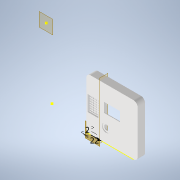
# Autodesk Inventor part: PCB_Deckel
Saved by Autodesk Inventor 2022.2 (Build 262287010, 287A)
## iProperties
Created: 2022-02-22
Part Number: PCB_Deckel
Material: Generisch
Document SubType Name: Modeling
Designer: hpcwoess
Density: 1 g/cm^3
Appearance: Vorgabe
Author: hpcwoess
Autodesk Inventor part; units mm, degrees
ref_plane "YZ Plane" through (0, 0, 0) normal (1, 0, 0) x (0, 1, 0)
ref_plane "XZ Plane" through (0, 0, 0) normal (0, 1, 0) x (-1, 0, 0)
ref_plane "Arbeitsebene1" through (0, 0, 9) normal (0, 0, 1) x (1, 0, 0)
sketch "Skizze1" plane through (0, 0, 9) normal (0, 0, 1) x (1, 0, 0)
  line L0 (68, -33.7) -> (131, -33.7)
  arc A0 (135.4, -38.1) -> (131, -33.7) centre (131, -38.1) ccw
  line L1 (135.4, -38.1) -> (135.4, -101.1)
  arc A1 (131, -105.5) -> (135.4, -101.1) centre (131, -101.1) ccw
  line L2 (131, -105.5) -> (68, -105.5)
  arc A2 (63.6, -101.1) -> (68, -105.5) centre (68, -101.1) ccw
  line L3 (63.6, -101.1) -> (63.6, -38.1)
  arc A3 (68, -33.7) -> (63.6, -38.1) centre (68, -38.1) ccw
  line L4 (131, -31.7) -> (68, -31.7)
  arc A4 (68, -31.7) -> (61.6, -38.1) centre (68, -38.1) ccw
  line L5 (61.6, -38.1) -> (61.6, -101.1)
  arc A5 (61.6, -101.1) -> (68, -107.5) centre (68, -101.1) ccw
  line L6 (68, -107.5) -> (131, -107.5)
  arc A6 (131, -107.5) -> (137.4, -101.1) centre (131, -101.1) ccw
  line L7 (137.4, -101.1) -> (137.4, -38.1)
  arc A7 (137.4, -38.1) -> (131, -31.7) centre (131, -38.1) ccw
  circle A8 centre (90.798, -87.67) radius 3.75
  line L8 (87.5, -55.7) -> (111.5, -55.7)
  line L9 (111.5, -55.7) -> (111.5, -69.7)
  line L10 (111.5, -69.7) -> (87.5, -69.7)
  line L11 (87.5, -69.7) -> (87.5, -55.7)
  circle A9 centre (73.806, -50.504) radius 4.35
  circle A10 centre (73.806, -87.588) radius 4.35
  point P0 (0, 0)
  point P1 (99.5, -55.7)
  dimension "d2" = 2
  dimension "d3" = 7.5
  dimension "d6" = 24
  dimension "d7" = 14
  dimension "d8" = 71.8
  dimension "d9" = 23.9
  dimension "d10" = 22
  constraints: 24 end point, 16 point on circle, 11 centre point, 2 parallel, 1 horizontal, 1 midpoint, 1 perpendicular, 7 other
  measures "d2" distance between parallel lines of L0 L4
  measures "d3" diameter of A8
  measures "d6" distance of L9.end L10.end
  measures "d7" distance of L8.end L9.end
  measures "d8" distance between parallel lines of L1 L3
  measures "d9" distance between parallel lines of L11 L3
  measures "d10" distance from line of point (99.5, -55.7) L0
extrude "Extrusion1" add sketch "Skizze1" along normal blind 2 contours L0 A0 L1 A1 L2 A2 L3 A3 | A7 L7 A6 L6 A5 L5 A4 L4 | A9 | A10
sketch "Skizze2" plane through (0, 0, 9) normal (0, 0, -1) x (-1, 0, 0)
  line L0 (-61.6, -38.1) -> (-61.6, -101.1) projected
  arc A0 (-61.6, -38.1) -> (-68, -31.7) centre (-68, -38.1) ccw projected
  line L1 (-131, -31.7) -> (-68, -31.7) projected
  arc A1 (-131, -31.7) -> (-137.4, -38.1) centre (-131, -38.1) ccw projected
  line L2 (-137.4, -101.1) -> (-137.4, -38.1) projected
  arc A2 (-137.4, -101.1) -> (-131, -107.5) centre (-131, -101.1) ccw projected
  line L3 (-68, -107.5) -> (-131, -107.5) projected
  arc A3 (-68, -107.5) -> (-61.6, -101.1) centre (-68, -101.1) ccw projected
  line L4 (-63.6, -101.1) -> (-63.6, -38.1)
  arc A4 (-63.6, -38.1) -> (-68, -33.7) centre (-68, -38.1) ccw
  line L5 (-68, -33.7) -> (-131, -33.7)
  arc A5 (-131, -33.7) -> (-135.4, -38.1) centre (-131, -38.1) ccw
  line L6 (-135.4, -38.1) -> (-135.4, -101.1)
  arc A6 (-135.4, -101.1) -> (-131, -105.5) centre (-131, -101.1) ccw
  line L7 (-131, -105.5) -> (-68, -105.5)
  arc A7 (-68, -105.5) -> (-63.6, -101.1) centre (-68, -101.1) ccw
  point P0 (0, 0)
  dimension "d15" = 2
  constraints: 8 end point, 8 point on circle, 4 centre point, 7 other
  measures "d15" distance between parallel lines of L0 L4
extrude "Extrusion2" add sketch "Skizze2" along normal blind 9
sketch "Skizze3" plane through (87.5, -55.7, 9) normal (0, -1, 0) x (1, 0, 0)
  line L0 (-19.5, 0) -> (43.5, 0) projected
  line L1 (-5.6, 0) -> (-4, 0)
  line L2 (-4, 0) -> (-4, -7.3)
  line L3 (-4, -7.3) -> (-5.6, -7.3)
  line L4 (-5.6, -7.3) -> (-5.6, 0)
  line L5 (-23.9, 0) -> (-23.9, -9) projected
  point P0 (-87.5, -9)
  point P1 (-4, 0)
  dimension "d18" = 1.6
  dimension "d19" = 18.3
  dimension "d20" = 7.3
  constraints: 8 end point, 2 parallel, 1 horizontal, 1 perpendicular, 1 point on line
  measures "d18" distance of L2.end L3.end
  measures "d19" distance between parallel lines of L5 L4
  measures "d20" distance of L3.end L1.start
extrude "Extrusion3" add sketch "Skizze3" along normal blind 51.75 and the other way blind 24
sketch "Skizze4" plane through (0, 0, 9) normal (0, 0, -1) x (-1, 0, 0)
  line L0 (-131, -33.7) -> (-68, -33.7) projected
  arc A0 (-63.6, -38.1) -> (-68, -33.7) centre (-68, -38.1) ccw projected
  line L1 (-63.6, -38.1) -> (-63.6, -101.1) projected
  arc A1 (-68, -105.5) -> (-63.6, -101.1) centre (-68, -101.1) ccw projected
  line L2 (-68, -105.5) -> (-131, -105.5) projected
  line L3 (-81.9, -33.7) -> (-81.9, -105.5) projected
  line L4 (-81.9, -33.7) -> (-81.9, -105.5) projected
  line L5 (-81.9, -33.7) -> (-81.9, -105.5)
  line L6 (-81.9, -105.5) -> (-68, -105.5)
  line L7 (-63.6, -58.7) -> (-81.9, -58.7)
  line L8 (-63.6, -79.5) -> (-81.9, -79.5)
  circle A2 centre (-73.806, -50.504) radius 4.35 projected
  circle A3 centre (-73.806, -87.588) radius 4.35 projected
  point P0 (0, 0)
  dimension "d25" = 25
  dimension "d26" = 26
  constraints: 8 end point, 4 point on line, 2 perpendicular, 1 collinear, 1 vertical
  measures "d25" distance from line of L0 L7.end
  measures "d26" distance from line of L8.end L2
extrude "Extrusion4" add sketch "Skizze4" along normal blind 2.75 contours L0 A0 L1 L7 L3 | L8 L1 A1 L2 L3
sketch "Skizze5" plane through (0, 0, 6.25) normal (0, 0, -1) x (-1, 0, 0)
  line L0 (-81.9, -58.7) -> (-63.6, -58.7) projected
  line L1 (-81.9, -33.7) -> (-81.9, -105.5) projected
  line L2 (-63.6, -58.7) -> (-81.9, -58.7)
  line L3 (-81.9, -58.7) -> (-81.9, -56.7)
  line L4 (-81.9, -56.7) -> (-63.6, -56.7)
  line L5 (-63.6, -56.7) -> (-63.6, -58.7)
  line L6 (-63.6, -79.5) -> (-63.6, -101.1) projected
  line L7 (-63.6, -79.5) -> (-81.9, -79.5)
  line L8 (-81.9, -79.5) -> (-81.9, -81.5)
  line L9 (-81.9, -81.5) -> (-63.6, -81.5)
  line L10 (-63.6, -81.5) -> (-63.6, -79.5)
  point P0 (0, 0)
  dimension "d29" = 2
  dimension "d30" = 2
  constraints: 16 end point, 4 parallel, 2 horizontal, 2 perpendicular, 2 point on line
  measures "d29" distance between parallel lines of L9 L7
  measures "d30" distance between parallel lines of L0 L4
extrude "Extrusion5" add sketch "Skizze5" along normal up to surface (4.55 mm away)
sketch "Skizze6" plane through (68, -107.5, 11) normal (0, -1, 0) x (1, 0, 0)
  line L0 (-4.4, -4.75) -> (13.9, -4.75) projected
  line L1 (13.9, -4.75) -> (13.9, -4.75) projected
  line L2 (0, -4.75) -> (13.9, -4.75) projected
  line L3 (-4.4, -4.75) -> (0, -4.75) projected
  line L4 (-4.4, -4.75) -> (-4.4, -4.75) projected
  line L5 (10.156, -4.75) -> (1.456, -4.75) projected
  line L6 (-6.4, -11) -> (-6.4, 0) projected
  line L7 (-6.4, -2.75) -> (12.85, -2.75)
  line L8 (63, 0) -> (0, 0) projected
  arc A0 (12.85, -2.75) -> (15.6, 0) centre (12.85, 0) ccw
  line L9 (-6.4, -2.75) -> (-6.4, 0)
  line L10 (0, 0) -> (-6.4, 0) projected
  line L11 (15.6, 0) -> (0, 0)
  line L12 (0, 0) -> (63, 0) projected
  point P0 (-68, -11)
  point P1 (5.806, -4.75)
  dimension "d33" = 2
  dimension "d102" = 22
  constraints: 6 end point, 2 horizontal, 2 point on circle, 2 point on line, 1 centre point, 1 collinear, 1 line through centre, 1 midpoint, 1 tangent
  measures "d33" distance from line of L7 point (5.806, -4.75)
  measures "d102" distance from line of L11.start L6
ref_plane "Arbeitsebene2" through (81.9, -81.5, 1.7) normal (1, 0, 0) x (0, 1, 0)
sketch "Skizze9" plane through (81.9, -81.5, 1.7) normal (1, 0, 0) x (0, 1, 0)
  line L0 (-24, 0) -> (47.8, 0) projected
  line L1 (18.0018, 0) -> (13.8035, 0)
  line L2 (13.8035, 0) -> (13.8035, 1.2366)
  line L3 (13.8035, 1.2366) -> (18.0018, 1.2366)
  line L4 (18.0018, 1.2366) -> (18.0018, 0)
  line L5 (-16.9587, 0) -> (-21.7715, 0)
  line L6 (-21.7715, 0) -> (-21.7715, 0.4193)
  line L7 (-21.7715, 0.4193) -> (-16.9587, 0.4193)
  line L8 (-16.9587, 0.4193) -> (-16.9587, 0)
  point P0 (81.5, -1.7)
  constraints: 16 end point, 4 parallel, 2 horizontal, 2 perpendicular, 2 point on line
extrude "Extrusion8" cut sketch "Skizze9" along normal blind 10
ref_plane "Arbeitsebene4" through (68, -107.5, 8.25) normal (0, 0, 1) x (1, 0, 0)
sketch "Skizze10" plane through (68, -107.5, 11) normal (0, 0, 1) x (1, 0, 0)
  line L0 (-4.4, 69.4) -> (-4.4, 6.4) projected
  line L1 (-4.4, 49.8) -> (11.6, 49.8)
  line L2 (11.6, 49.8) -> (11.6, 26.8)
  line L3 (11.6, 26.8) -> (-4.4, 26.8)
  line L4 (-4.4, 26.8) -> (-4.4, 49.8)
  line L5 (12.85, 48.8) -> (-4.4, 48.8) projected
  point P0 (-68, 107.5)
  point P1 (13.9021, 48.8)
  point P2 (-4.4, 26.8)
  dimension "d43" = 16
  dimension "d44" = 23
  dimension "d45" = 1
  constraints: 8 end point, 2 parallel, 1 horizontal, 1 perpendicular, 1 point on line
  measures "d43" distance of L2.end L3.end
  measures "d44" distance of L1.end L2.end
  measures "d45" distance from line of L1.start L5
extrude "Extrusion9" cut sketch "Skizze10" against normal blind 2
ref_plane "Arbeitsebene3" through (68, -107.5, 8.25) normal (0, 0, 1) x (1, 0, 0)
sketch "Skizze11" plane through (68, -107.5, 11) normal (0, 0, 1) x (1, 0, 0)
  line L0 (11.6, 48.8) -> (13.9, 48.8) projected
  line L1 (13.9, 28) -> (11.6, 28) projected
  line L2 (12.5525, 48.8) -> (11.6, 48.8)
  line L3 (11.6, 48.8) -> (11.6, 28)
  line L4 (11.6, 28) -> (12.5525, 28)
  line L5 (12.5525, 28) -> (12.5525, 48.8)
  point P0 (-68, 107.5)
  point P1 (11.6, 48.8)
  point P2 (12.5525, 28)
  constraints: 8 end point, 2 parallel, 1 horizontal, 1 perpendicular, 1 point on line
extrude "Extrusion10" add sketch "Skizze11" against normal up to surface (9.3 mm away)
ref_plane "Arbeitsebene5" through (68, -107.5, 8.25) normal (0, 0, 1) x (1, 0, 0)
sketch "Skizze12" plane through (68, -107.5, 8.25) normal (0, 0, 1) x (1, 0, 0)
  line L0 (11.6, 49.8) -> (-4.4, 49.8) projected
  line L1 (-4.4, 26.8) -> (11.6, 26.8) projected
  line L2 (10.4, 49.8) -> (9.2, 49.8)
  line L3 (9.2, 49.8) -> (9.2, 26.8)
  line L4 (9.2, 26.8) -> (10.4, 26.8)
  line L5 (10.4, 26.8) -> (10.4, 49.8)
  line L6 (11.6, 49.8) -> (11.6, 26.8) projected
  line L7 (8, 49.8) -> (6.8, 49.8)
  line L8 (6.8, 49.8) -> (6.8, 26.8)
  line L9 (6.8, 26.8) -> (8, 26.8)
  line L10 (8, 26.8) -> (8, 49.8)
  line L11 (5.6, 49.8) -> (4.4, 49.8)
  line L12 (4.4, 49.8) -> (4.4, 26.8)
  line L13 (4.4, 26.8) -> (5.6, 26.8)
  line L14 (5.6, 26.8) -> (5.6, 49.8)
  line L15 (3.2, 49.8) -> (2, 49.8)
  line L16 (2, 49.8) -> (2, 26.8)
  line L17 (2, 26.8) -> (3.2, 26.8)
  line L18 (3.2, 26.8) -> (3.2, 49.8)
  line L19 (0.8, 49.8) -> (-0.4, 49.8)
  line L20 (-0.4, 49.8) -> (-0.4, 26.8)
  line L21 (-0.4, 26.8) -> (0.8, 26.8)
  line L22 (0.8, 26.8) -> (0.8, 49.8)
  line L23 (-1.6, 49.8) -> (-2.8, 49.8)
  line L24 (-2.8, 49.8) -> (-2.8, 26.8)
  line L25 (-2.8, 26.8) -> (-1.6, 26.8)
  line L26 (-1.6, 26.8) -> (-1.6, 49.8)
  line L27 (-4, 49.8) -> (-5.2, 49.8)
  line L28 (-5.2, 49.8) -> (-5.2, 26.8)
  line L29 (-5.2, 26.8) -> (-4, 26.8)
  line L30 (-4, 26.8) -> (-4, 49.8)
  point P0 (-68, 107.5)
  point P1 (-1.6, 49.8)
  point P2 (-2.8, 49.8)
  point P3 (-2.8, 26.8)
  point P4 (0.8, 26.8)
  point P5 (0.8, 49.8)
  point P6 (-0.4, 49.8)
  point P7 (-0.4, 26.8)
  point P8 (3.2, 26.8)
  point P9 (3.2, 49.8)
  point P10 (2, 49.8)
  point P11 (2, 26.8)
  point P12 (5.6, 26.8)
  point P13 (5.6, 49.8)
  point P14 (4.4, 49.8)
  point P15 (4.4, 26.8)
  point P16 (8, 49.8)
  point P17 (6.8, 49.8)
  point P18 (6.8, 26.8)
  point P19 (10.4, 26.8)
  point P20 (9.2, 49.8)
  dimension "d50" = 1.2
  dimension "d51" = 1.2
  dimension "d54" = 2.4
  constraints: 56 end point, 2 horizontal, 2 parallel, 2 point on line, 1 perpendicular, 48 other
  measures "d50" distance between parallel lines of L3 L5
  measures "d51" distance between parallel lines of L5 L6
  measures "d54" distance of L2.start L7.start
extrude "Extrusion11" add sketch "Skizze12" against normal blind 1.4 contours L5 L1 L3 L0 | L10 L1 L8 L0 | L14 L1 L12 L0 | L18 L1 L16 L0 | L22 L1 L20 L0 | L26 L1 L24 L0
ref_plane "Arbeitsebene6" through (68, -107.5, 8.25) normal (0, 0, 1) x (1, 0, 0)
sketch "Skizze13" plane through (68, -107.5, 8.25) normal (0, 0, 1) x (1, 0, 0)
  line L0 (-4.4, 69.4) -> (-4.4, 6.4) projected
  line L1 (-4.4, 47.9612) -> (14.3855, 47.9612)
  line L2 (14.3855, 47.9612) -> (14.3855, 46.7612)
  line L3 (14.3855, 46.7612) -> (-4.4, 46.7612)
  line L4 (-4.4, 46.7612) -> (-4.4, 47.9612)
  line L5 (-4.4, 44.9612) -> (14.3855, 44.9612)
  line L6 (14.3855, 44.9612) -> (14.3855, 43.7612)
  line L7 (14.3855, 43.7612) -> (-4.4, 43.7612)
  line L8 (-4.4, 43.7612) -> (-4.4, 44.9612)
  line L9 (-4.4, 41.9612) -> (14.3855, 41.9612)
  line L10 (14.3855, 41.9612) -> (14.3855, 40.7612)
  line L11 (14.3855, 40.7612) -> (-4.4, 40.7612)
  line L12 (-4.4, 40.7612) -> (-4.4, 41.9612)
  line L13 (-4.4, 38.9612) -> (14.3855, 38.9612)
  line L14 (14.3855, 38.9612) -> (14.3855, 37.7612)
  line L15 (14.3855, 37.7612) -> (-4.4, 37.7612)
  line L16 (-4.4, 37.7612) -> (-4.4, 38.9612)
  line L17 (-4.4, 35.9612) -> (14.3855, 35.9612)
  line L18 (14.3855, 35.9612) -> (14.3855, 34.7612)
  line L19 (14.3855, 34.7612) -> (-4.4, 34.7612)
  line L20 (-4.4, 34.7612) -> (-4.4, 35.9612)
  line L21 (-4.4, 32.9612) -> (14.3855, 32.9612)
  line L22 (14.3855, 32.9612) -> (14.3855, 31.7612)
  line L23 (14.3855, 31.7612) -> (-4.4, 31.7612)
  line L24 (-4.4, 31.7612) -> (-4.4, 32.9612)
  line L25 (-4.4, 29.9612) -> (14.3855, 29.9612)
  line L26 (14.3855, 29.9612) -> (14.3855, 28.7612)
  line L27 (14.3855, 28.7612) -> (-4.4, 28.7612)
  line L28 (-4.4, 28.7612) -> (-4.4, 29.9612)
  point P0 (-68, 107.5)
  point P1 (-4.4, 29.9612)
  point P2 (-4.4, 28.7612)
  point P3 (-4.4, 32.9612)
  point P4 (-4.4, 31.7612)
  point P5 (-4.4, 35.9612)
  point P6 (-4.4, 34.7612)
  point P7 (-4.4, 38.9612)
  point P8 (-4.4, 37.7612)
  point P9 (-4.4, 41.9612)
  point P10 (-4.4, 40.7612)
  point P11 (-4.4, 44.9612)
  point P12 (-4.4, 43.7612)
  point P13 (-4.4, 46.7612)
  dimension "d61" = 1.2
  dimension "d64" = 3
  constraints: 56 end point, 2 parallel, 1 horizontal, 1 perpendicular, 1 point on line, 49 other
  measures "d61" distance between parallel lines of L3 L1
  measures "d64" distance of L1.start L5.start
extrude "Extrusion12" add sketch "Skizze13" against normal blind 1.4
sketch "Skizze14" plane through (61.6, -101.1, 0) normal (-1, 0, 0) x (0, 0, 1)
  line L0 (4.6329, 43.4) -> (2.6329, 43.4)
  line L1 (2.6329, 43.4) -> (2.6329, 19.6)
  line L2 (2.6329, 19.6) -> (4.6329, 19.6)
  line L3 (4.6329, 19.6) -> (4.6329, 43.4)
  line L4 (8.25, 43.4) -> (1.7, 43.4) projected
  line L5 (1.7, 19.6) -> (6.25, 19.6) projected
  point P0 (0, 101.1)
  point P1 (4.6329, 31.5)
  dimension "d71" = 2
  dimension "d72" = 0
  dimension "d73" = 0
  constraints: 8 end point, 2 parallel, 1 horizontal, 1 midpoint, 1 perpendicular
  measures "d71" distance from line of L1 point (4.633, 31.5)
  measures "d72" distance between parallel lines of L4 L0
  measures "d73" distance between parallel lines of L5 L2
extrude "Extrusion13" cut sketch "Skizze14" against normal blind 2.9
sketch "Skizze15" plane through (0, 0, 9) normal (0, 0, -1) x (-1, 0, 0)
  line L0 (-113, -49.7) -> (-86, -49.7)
  line L1 (-86, -49.7) -> (-86, -76.7)
  line L2 (-86, -76.7) -> (-113, -76.7)
  line L3 (-113, -76.7) -> (-113, -49.7)
  line L4 (-84, -47.7) -> (-115, -47.7)
  line L5 (-115, -47.7) -> (-115, -78.7)
  line L6 (-115, -78.7) -> (-84, -78.7)
  line L7 (-84, -78.7) -> (-84, -47.7)
  line L8 (-87.5, -55.7) -> (-111.5, -55.7) projected
  line L9 (-111.5, -69.7) -> (-87.5, -69.7) projected
  point P0 (0, 0)
  point P1 (-99.5, -47.7)
  point P2 (-99.5, -55.7)
  dimension "d76" = 2
  dimension "d77" = 27
  dimension "d78" = 0
  dimension "d79" = 7
  dimension "d80" = 27
  constraints: 16 end point, 4 parallel, 2 midpoint, 2 perpendicular, 1 horizontal, 3 other
  measures "d76" distance between parallel lines of L0 L4
  measures "d77" distance between parallel lines of L1 L3
  measures "d78" horizontal distance of point (-99.5, -47.7) point (-99.5, -55.7)
  measures "d79" distance between parallel lines of L9 L2
  measures "d80" distance between parallel lines of L0 L2
extrude "Extrusion14" add sketch "Skizze15" along normal blind 3.5
sketch "Skizze16" plane through (81.9, -56.7, 1.7) normal (0, 0, -1) x (-1, 0, 0)
  line L0 (2.3, -1) -> (-3.6265, -1)
  line L1 (-3.6265, -1) -> (-3.6265, -4.4021)
  line L2 (-3.6265, -4.4021) -> (2.3, -4.4021)
  line L3 (2.3, -4.4021) -> (2.3, -1)
  point P0 (81.9, 56.7)
  constraints: 8 end point, 2 parallel, 1 horizontal, 1 perpendicular
extrude "Extrusion15" cut sketch "Skizze16" against normal blind 3.5
sketch "Skizze17" plane through (0, 0, 9) normal (0, 0, -1) x (-1, 0, 0)
  line L0 (-83.5, -33.7) -> (-131, -33.7) projected
  arc A0 (-131, -33.7) -> (-135.4, -38.1) centre (-131, -38.1) ccw projected
  line L1 (-129.8047, -33.7) -> (-134.6878, -33.7)
  line L2 (-134.6878, -33.7) -> (-134.6878, -35.7)
  line L3 (-134.6878, -35.7) -> (-129.8047, -35.7)
  line L4 (-129.8047, -35.7) -> (-129.8047, -33.7)
  line L5 (-131, -105.5) -> (-83.5, -105.5) projected
  arc A1 (-135.4, -101.1) -> (-131, -105.5) centre (-131, -101.1) ccw projected
  line L6 (-129.8047, -105.5) -> (-134.6878, -105.5)
  line L7 (-134.6878, -105.5) -> (-134.6878, -103.5)
  line L8 (-134.6878, -103.5) -> (-129.8047, -103.5)
  line L9 (-129.8047, -103.5) -> (-129.8047, -105.5)
  point P0 (0, 0)
  point P1 (-84.0221, -33.7)
  point P2 (-84.0221, -105.5)
  point P3 (-129.8047, -105.5)
  point P4 (-129.8047, -33.7)
  dimension "d85" = 2
  constraints: 16 end point, 4 parallel, 4 point on line, 2 horizontal, 2 perpendicular, 2 point on circle
  measures "d85" distance of L2.end L1.end
extrude "Extrusion16" add sketch "Skizze17" along normal up to surface (7.3 mm away)
sketch "Skizze18" plane through (0, 0, 11) normal (0, 0, 1) x (1, 0, 0)
  circle A0 centre (90.798, -87.67) radius 3.75 projected
  circle A1 centre (90.798, -87.67) radius 6
  point P0 (0, 0)
  dimension "d88" = 12
  constraints: 1 centre point, 1 coincident
  measures "d88" diameter of A1
sketch "Skizze19" plane through (0, 0, 9) normal (0, 0, -1) x (-1, 0, 0)
  line L0 (-100.398, -86.4566) -> (-96.398, -86.4566)
  line L1 (-96.398, -86.4566) -> (-96.398, -88.9566)
  line L2 (-96.398, -88.9566) -> (-100.398, -88.9566)
  line L3 (-100.398, -88.9566) -> (-100.398, -86.4566)
  circle A0 centre (-90.798, -87.67) radius 3.75 projected
  point P0 (0, 0)
  point P1 (-98.398, -88.9566)
  point P2 (-98.398, -86.4566)
  dimension "d89" = 2.5
  dimension "d90" = 4
  dimension "d91" = 7.6
  constraints: 8 end point, 2 midpoint, 2 parallel, 1 horizontal, 1 perpendicular
  measures "d89" distance of point (-98.398, -88.957) point (-98.398, -86.457)
  measures "d90" distance between parallel lines of L1 L3
  measures "d91" horizontal distance of A0.centre point (-98.398, -88.957)
extrude "Extrusion17" cut sketch "Skizze19" against normal blind 1.4 contours L0 L1 L2 L3
extrude "Extrusion18" cut sketch "Skizze18" against normal blind 1
sketch "Skizze20" plane through (0, 0, 9) normal (0, 0, -1) x (-1, 0, 0)
  line L0 (-86, -49.7) -> (-86, -76.7) projected
  line L1 (-113, -76.7) -> (-113, -49.7) projected
  line L2 (-86, -73.7) -> (-113, -73.7)
  line L3 (-113, -73.7) -> (-113, -52.7)
  line L4 (-113, -52.7) -> (-86, -52.7)
  line L5 (-86, -52.7) -> (-86, -73.7)
  line L6 (-86, -76.7) -> (-113, -76.7) projected
  line L7 (-113, -49.7) -> (-86, -49.7) projected
  line L8 (-110, -52.7) -> (-89, -52.7)
  line L9 (-89, -52.7) -> (-89, -49.7)
  line L10 (-89, -49.7) -> (-110, -49.7)
  line L11 (-110, -49.7) -> (-110, -52.7)
  point P0 (0, 0)
  point P1 (-110, -51.2)
  point P2 (-89, -51.2)
  dimension "d96" = 3
  dimension "d97" = 3
  dimension "d100" = 3
  dimension "d101" = 3
  constraints: 16 end point, 4 parallel, 4 point on line, 2 horizontal, 2 midpoint, 2 perpendicular
  measures "d96" distance between parallel lines of L2 L6
  measures "d97" distance between parallel lines of L7 L4
  measures "d100" distance from line of point (-110, -51.2) L1
  measures "d101" distance from line of L0 point (-89, -51.2)
extrude "Extrusion19" cut sketch "Skizze20" against normal blind 1 contours L0 L2 L1 L4 | L9 L4 L11 L7
sketch "Skizze21" plane through (68, -107.5, 8.25) normal (0, 0, 1) x (1, 0, 0)
  point P0 (-68, 107.5)
equation "\"d9\" = -0.5 * d6 + 0.5 * d8"
equation "\"d30\" = d29"
equation "\"d51\" = d50"
equation "\"d101\" = d100"
